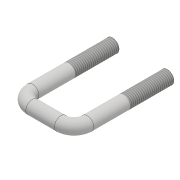
# Autodesk Inventor part: Suspension_Clamp_U-Bolt
Saved by Autodesk Inventor 2018 (Build 220112000, 112)
## iProperties
Created: 2021-04-28
Part Number: Suspension_Clamp_U-Bolt
Material: Generic
Document SubType Name: Modeling
Designer: l01767
Density: 1 g/cm^3
Appearance: Default
Author: l01767
Autodesk Inventor part; units mm, degrees
ref_plane "YZ Plane" through (0, 0, 0) normal (1, 0, 0) x (0, 1, 0)
ref_plane "XZ Plane" through (0, 0, 0) normal (0, 1, 0) x (-1, 0, 0)
ref_plane "XY Plane" through (0, 0, 0) normal (0, 0, 1) x (1, 0, 0)
sketch "Sketch1" plane through (0, 0, 0) normal (1, 0, 0) x (0, 1, 0)
  circle A0 centre (0, 0) radius 6
  dimension "d0" = 12
  constraints: 1 centre point, 1 coincident
  measures "d0" diameter of A0
sketch "Sketch2" plane through (0, 0, 0) normal (0, 0, 1) x (1, 0, 0)
  line L0 (0, 0) -> (13, 0)
  line L1 (25, 12) -> (25, 85)
  line L2 (0, 0) -> (0, 120)
  line L3 (0, 0) -> (-13, 0)
  line L4 (-25, 12) -> (-25, 85)
  arc A0 (-25, 12) -> (-13, 0) centre (-13, 12) ccw
  arc A1 (13, 0) -> (25, 12) centre (13, 12) ccw
  point P0 (25, 0)
  point P1 (-25, 0)
  dimension "d1" = 25
  dimension "d2" = 85
  dimension "d3" = 12
  constraints: 10 end point, 4 point on circle, 4 point on line, 4 tangent, 2 centre point, 2 symmetric about line, 1 equal radius, 1 horizontal, 1 perpendicular, 1 vertical
  measures "d1" distance of L0.start point (25, 0)
  measures "d2" distance of point (25, 0) L1.end
  measures "d3" radius of A0
sweep "Sweep1" add profiles "Sketch1" path "Sketch2" path curves L1 A1 L0 L3 A0 L4
thread "Thread1"
thread "Thread2"
body "Solid1"
